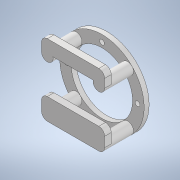
# Autodesk Inventor part: Soporte_Servo
Saved by Autodesk Inventor 2020.1 (Build 241239000, 239)
## iProperties
Created: 2019-12-05
Part Number: Soporte_Servo
Material: Generic
Document SubType Name: Modeling
Designer: Daniel
Density: 1 g/cm^3
Appearance: Default
Author: Daniel
Autodesk Inventor part; units mm, degrees
ref_plane "YZ Plane" through (0, 0, 0) normal (1, 0, 0) x (0, 1, 0)
ref_plane "XZ Plane" through (0, 0, 0) normal (0, 1, 0) x (-1, 0, 0)
ref_plane "XY Plane" through (0, 0, 0) normal (0, 0, 1) x (1, 0, 0)
sketch "Sketch1" plane through (0, 0, 0) normal (0, 0, 1) x (1, 0, 0)
  circle A0 centre (-21.5, 0) radius 1.25 projected
  circle A1 centre (21.5, 0) radius 1.25 projected
  circle A2 centre (0, 21.5) radius 1.25 projected
  circle A3 centre (0, -21.5) radius 1.25 projected
  circle A4 centre (0, 0) radius 25.5 projected
  circle A5 centre (0, 0) radius 17.5 projected
  circle A6 centre (0, 0) radius 18.5
  circle A7 centre (0, 21.5) radius 1.45
  circle A8 centre (-21.5, 0) radius 1.45
  circle A9 centre (0, -21.5) radius 1.45
  circle A10 centre (21.5, 0) radius 1.45
  dimension "d0" = 1
  dimension "d3" = 0.2
  dimension "d6" = 360
  constraints: 5 centre point, 2 coincident, 9 other
  measures "d0" radial gap between concentric circles of A5 A6
  measures "d3" radial gap between concentric circles of A7 A2
extrude "Extrusion1" add sketch "Sketch1" along normal blind 3 contours A4
sketch "Sketch2" plane through (0, 0, 3) normal (0, 0, 1) x (1, 0, 0)
  circle A0 centre (0, 21.5) radius 1.45 construction
  line L0 (0, 0) -> (15.5563, 15.5563) construction
  line L1 (0, 0) -> (38.5383, 0) construction
  circle A1 centre (0, 0) radius 25.5 projected
  line L2 (-25.5, 0) -> (-18.5, 0) construction
  circle A2 centre (0, 0) radius 18.5 projected
  circle A3 centre (0, 0) radius 22 construction
  circle A4 centre (15.5563, 15.5563) radius 3.5
  circle A5 centre (-15.5563, 15.5563) radius 3.5
  circle A6 centre (-15.5563, -15.5563) radius 3.5
  circle A7 centre (15.5563, -15.5563) radius 3.5
  dimension "d9" = 44
  dimension "d8" = 45
  dimension "d12" = 360
  constraints: 6 end point, 4 centre point, 3 coincident, 2 horizontal, 2 horizontal alignment, 14 other
  measures "d8" angle of L1 L0
extrude "Extrusion2" add sketch "Sketch2" along normal blind 17.45 contours A4 | A7 | A5 | A6
sketch "Sketch3" plane through (15.5563, 15.5563, 20.45) normal (0, 0, 1) x (1, 0, 0)
  line L0 (-10.3063, -21.6563) -> (-20.8063, -21.6563) projected
  line L1 (-20.8063, 0.8437) -> (-10.3063, 0.8437) projected
  arc A0 (-28.6378, -2.4749) -> (-33.5876, 2.4749) centre (-31.1127, 0) ccw projected
  line L2 (-27.7159, 0.8437) -> (-3.3968, 0.8437)
  line L3 (3.5, -21.6563) -> (-34.6127, -21.6563)
  line L4 (3.5, -21.6563) -> (3.5, -31.1127)
  line L5 (0, -34.6127) -> (-31.1127, -34.6127)
  line L6 (-34.6127, -31.1127) -> (-34.6127, -21.6563)
  circle A1 centre (0, -31.1127) radius 3.5 projected
  circle A2 centre (-31.1127, -31.1127) radius 3.5 projected
  circle A3 centre (0, -31.1127) radius 3.5 projected
  circle A4 centre (-31.1127, -31.1127) radius 3.5 projected
  line L7 (3.5, 0) -> (3.5, 8.6437)
  line L8 (3.5, 8.6437) -> (-34.6127, 8.6437)
  line L9 (-34.6127, 8.6437) -> (-34.6127, 0)
  circle A5 centre (-31.1127, 0) radius 3.5 projected
  circle A6 centre (0, 0) radius 3.5 projected
  line L10 (-20.8063, 5.6437) -> (-16.1063, 5.6437) projected
  point P0 (-15.5563, -15.5563)
  point P1 (0, -34.6127)
  point P2 (-10.3063, 0.8437)
  dimension "d16" = 3
  constraints: 16 end point, 8 point on circle, 5 tangent, 4 perpendicular, 2 collinear, 2 horizontal, 2 vertical
  measures "d16" distance between parallel lines of L8 L10
extrude "Extrusion3" add sketch "Sketch3" against normal blind 4
fillet "Fillet1" radius 3.5 4 edges at (19.0563, 24.2, 18.45) (19.0563, -6.1, 18.45) (-19.0563, -6.1, 18.45) (-19.0563, 24.2, 18.45)
body "Solid1"
